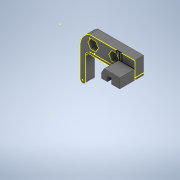
# Autodesk Inventor part: mount_battery
Saved by Autodesk Inventor 2022.2 (Build 262287000, 287)
## iProperties
Created: 2021-01-30
Part Number: mount_battery
Material: ABS Plastic
Document SubType Name: Modeling
Designer: User
Density: 1.06 g/cm^3
Appearance: Smooth - Black
Author: User
Autodesk Inventor part; units mm, degrees
ref_plane "YZ Plane" through (0, 0, 0) normal (1, 0, 0) x (0, 1, 0)
ref_plane "XZ Plane" through (0, 0, 0) normal (0, 1, 0) x (-1, 0, 0)
ref_plane "Work Plane1" through (0, 0, 0) normal (0, 0, 1) x (1, 0, 0)
sketch "mount_sketch" plane through (0, 0, 0) normal (0, 0, 1) x (1, 0, 0)
  circle A0 centre (42, 55.2584) radius 1.55 projected
  circle A1 centre (28, 55.2584) radius 1.55 projected
  line L0 (45, 60.2584) -> (25, 60.2584)
  line L1 (25, 60.2584) -> (15.4, 52.7584)
  line L2 (15.4, 52.7584) -> (15.4, 29.5584)
  line L3 (15.4, 29.5584) -> (19.4, 29.5584)
  line L4 (19.4, 29.5584) -> (19.4, 48.7584)
  line L5 (19.4, 48.7584) -> (23, 48.7584)
  circle A2 centre (42, -54.7416) radius 1.55 construction
  circle A3 centre (28, -54.7416) radius 1.55 construction
  line L6 (47, -54.627) -> (47, 66.2497) construction
  circle A4 centre (12, 51.2584) radius 1.55 construction
  circle A5 centre (12, -37.8416) radius 1.55 construction
  circle A6 centre (12, -54.7416) radius 1.55 construction
  circle A7 centre (29, -68.7416) radius 1.55 construction
  circle A8 centre (14, -68.7416) radius 1.55 construction
  line L7 (45, 50.2584) -> (25, 50.2584)
  line L8 (25, 50.2584) -> (23, 48.7584)
  line L9 (45, 60.2584) -> (46.5, 60.2584)
  line L10 (46.5, 60.2584) -> (46.5, 50.2584)
  line L11 (46.5, 50.2584) -> (45, 50.2584)
  line L12 (23, 48.7584) -> (23, 58.6959)
  line L13 (35, 55.2584) -> (35, 60.2584)
  line L14 (35, 55.2584) -> (35, 50.2584)
  line L15 (46.5, 60.2584) -> (50, 60.2584)
  line L16 (50, 60.2584) -> (50, 50.2584)
  line L17 (50, 50.2584) -> (46.5, 50.2584)
  line L18 (50, 60.2584) -> (56, 60.2584)
  line L19 (56, 60.2584) -> (56, 50.2584)
  line L20 (56, 50.2584) -> (50, 50.2584)
  line L21 (53, 50.2584) -> (56, 50.2584)
  line L22 (53, 50.2584) -> (53, 60.2584)
  point P0 (0, 0)
  dimension "d1" = 110
  dimension "d2" = 6.5
  dimension "d3" = 27.6
  dimension "d4" = 4
  dimension "d5" = 14
  dimension "d6" = 5
  dimension "d7" = 19.2
  dimension "d9" = 3.4
  dimension "d13" = 3
  dimension "d30" = 2
  dimension "d32" = 5
  dimension "d62" = 4.5
  dimension "d77" = 8
  dimension "d78" = 6
  constraints: 44 end point, 11 perpendicular, 4 horizontal, 4 midpoint, 2 vertical alignment, 1 collinear, 1 point on line, 1 vertical
  measures "d1" distance of A2.centre A0.centre
  measures "d2" distance from line of A0.centre L5
  measures "d3" distance between parallel lines of L6 L4
  measures "d4" distance between parallel lines of L4 L2
  measures "d5" vertical distance of A3.centre A7.centre
  measures "d6" distance from line of L0 A0.centre
  measures "d7" distance between parallel lines of L5 L3
  measures "d9" distance from line of L2 A4.centre
  measures "d13" horizontal distance of L0.end A1.centre
  measures "d30" horizontal distance of L0.end L5.end
  measures "d32" distance from line of L7 A0.centre
  measures "d62" distance from line of L10 A0.centre
  measures "d77" distance from line of L16 A0.centre
  measures "d78" distance of L19.end L16.end
extrude "mount" add sketch "mount_sketch" along normal blind 6 contours L9 L10 L11 L7 L14 L13 L0 | L13 L14 L7 L8 L12 L1 L0 | L12 L5 L4 L3 L2 L1
fillet "common" radius 2 2 edges at (25, 60.2584, 3) (25, 50.2584, 3)
sketch "nuts_sketch" plane through (0, 0, 6) normal (0, 0, 1) x (1, 0, 0)
  circle A0 centre (42, 55.2584) radius 1.55 projected
  circle A1 centre (28, 55.2584) radius 1.55 projected
  line L0 (38.4782, 55.2584) -> (40.2391, 58.3084)
  line L1 (40.2391, 58.3084) -> (43.7609, 58.3084)
  line L2 (43.7609, 58.3084) -> (45.5218, 55.2584)
  line L3 (45.5218, 55.2584) -> (43.7609, 52.2084)
  line L4 (43.7609, 52.2084) -> (40.2391, 52.2084)
  line L5 (40.2391, 52.2084) -> (38.4782, 55.2584)
  line L6 (31.5218, 55.2584) -> (29.7609, 52.2084)
  line L7 (29.7609, 52.2084) -> (26.2391, 52.2084)
  line L8 (26.2391, 52.2084) -> (24.4782, 55.2584)
  line L9 (24.4782, 55.2584) -> (26.2391, 58.3084)
  line L10 (26.2391, 58.3084) -> (29.7609, 58.3084)
  line L11 (29.7609, 58.3084) -> (31.5218, 55.2584)
  point P0 (0, 0)
  dimension "d26" = 6.1
  dimension "d27" = 6.1
  constraints: 24 end point, 2 coincident, 2 horizontal alignment, 26 other
  measures "d26" distance between parallel lines of L2 L5
  measures "d27" distance between parallel lines of L8 L11
extrude "nuts" cut sketch "nuts_sketch" against normal blind 3
sketch "Sketch11" plane through (25.6667, 50.2584, 0) normal (0, -1, 0) x (1, 0, 0)
  point P0 (-25.6667, 0)
  point P1 (12.8115, -12)
sketch "Sketch13" plane through (46.5, 50.2584, 0) normal (1, 0, 0) x (0, 0, -1)
  line L0 (0, 10) -> (-6, 10) projected
  line L1 (0, 0) -> (-6, 0) projected
  line L2 (-6, 10) -> (-6, 0)
  line L3 (0, 0) -> (0, 10) projected
  line L4 (-6, 0) -> (0, 0)
  line L5 (0, 0) -> (0, 10)
  line L6 (0, 10) -> (-6, 10)
  point P0 (0, -50.2584)
  constraints: 8 end point, 3 perpendicular, 1 vertical
extrude "Extrusion11" add sketch "Sketch13" along normal blind 9.5
sketch "Sketch20" plane through (19.4, 29.5584, 0) normal (1, 0, 0) x (0, 0, -1)
  line L0 (-6, 0) -> (-6, 19.2) projected
  line L1 (-6, 0) -> (-6, 19.2)
  line L2 (0, 19.2) -> (-6, 19.2) projected
  line L3 (-6, 19.2) -> (0, 19.2)
  line L4 (0, 0) -> (-6, 0) projected
  line L5 (0, 19.2) -> (0, 0)
  line L6 (0, 0) -> (-6, 0)
  point P0 (0, -29.5584)
  constraints: 8 end point, 2 collinear, 1 perpendicular, 1 vertical
extrude "Extrusion15" add sketch "Sketch20" along normal blind 3.6
sketch "Sketch21" plane through (0, 0, 6) normal (0, 0, 1) x (1, 0, 0)
  line L0 (15.4, 29.5584) -> (23, 29.5584) projected
  line L1 (19.2, 29.5584) -> (19.2, 55.7272)
  line L2 (24.4573, 59.8345) -> (15.4, 52.7584) projected
  line L3 (15.4, 52.7584) -> (15.4, 29.5584) projected
  line L4 (19.2, 29.5584) -> (15.4, 29.5584)
  line L5 (15.4, 29.5584) -> (15.4, 52.7584)
  line L6 (15.4, 52.7584) -> (19.2, 55.7272)
  line L7 (23, 48.7584) -> (24.4667, 49.8584) projected
  line L8 (23, 48.7584) -> (19.2, 48.7584)
  line L9 (23, 48.7584) -> (23, 29.5584) projected
  line L10 (23, 48.7584) -> (23, 58.6959)
  line L11 (19.2, 48.7584) -> (23, 58.6959)
  point P0 (0, 0)
  constraints: 14 end point, 3 point on line, 2 vertical, 1 collinear, 1 horizontal, 1 midpoint, 1 perpendicular
extrude "Extrusion16" cut sketch "Sketch21" against normal blind 6 contours L3 L2 L1 L0
sketch "Sketch22" plane through (0, 0, 6) normal (0, 0, 1) x (1, 0, 0)
  line L0 (23, 48.7584) -> (23, 29.5584) projected
  line L1 (23, 48.7584) -> (23, 58.6959)
  line L2 (24.4573, 59.8345) -> (19.2, 55.7272) projected
  line L3 (23, 48.7584) -> (19.2, 48.7584)
  line L4 (19.2, 29.5584) -> (19.2, 55.7272) projected
  point P0 (0, 0)
  constraints: 4 end point, 2 point on line, 1 perpendicular, 1 vertical
fillet "Fillet12" radius 10 1 edges at (19.2, 55.7272, 3)
fillet "Fillet13" radius 2 1 edges at (23, 48.7584, 3)
fillet "Fillet14" radius 2 2 edges at (23, 29.5584, 3) (19.2, 29.5584, 3)
sketch "Sketch27" plane through (25.6667, 50.2584, 0) normal (0, -1, 0) x (1, 0, 0)
  line L0 (0, 0) -> (0, 6) projected
  line L1 (0, 0) -> (30.3333, 0) projected
  line L2 (30.3333, 6) -> (30.3333, 0) projected
  line L3 (0, 6) -> (30.3333, 6) projected
  point P0 (-25.6667, 0)
extrude "Extrusion21" add sketch "Sketch27" along normal blind 1.5
sketch "Sketch28" plane through (25.6667, 48.7584, 0) normal (-1, 0, 0) x (0, 0, 1)
  line L0 (0, 1.5) -> (6, 1.5) projected
  line L1 (0, 1.5) -> (0, 0) projected
  line L2 (6, 0) -> (0, 0) projected
  line L3 (6, 1.5) -> (6, 0) projected
  point P0 (0, -48.7584)
extrude "Extrusion22" add sketch "Sketch28" along normal through all
fillet "Fillet19" radius 1 1 edges at (23.2679, 48.7584, 3)
sketch "Sketch29" plane through (0, 0, 6) normal (0, 0, 1) x (1, 0, 0)
  line L0 (24.4782, 55.2584) -> (26.2391, 58.3084) projected
  line L1 (26.2391, 58.3084) -> (29.7609, 58.3084) projected
  line L2 (29.7609, 58.3084) -> (31.5218, 55.2584) projected
  line L3 (31.5218, 55.2584) -> (29.7609, 52.2084) projected
  line L4 (29.7609, 52.2084) -> (26.2391, 52.2084) projected
  line L5 (26.2391, 52.2084) -> (24.4782, 55.2584) projected
  line L6 (45.5218, 55.2584) -> (43.7609, 52.2084) projected
  line L7 (43.7609, 52.2084) -> (40.2391, 52.2084) projected
  line L8 (40.2391, 52.2084) -> (38.4782, 55.2584) projected
  line L9 (38.4782, 55.2584) -> (40.2391, 58.3084) projected
  line L10 (40.2391, 58.3084) -> (43.7609, 58.3084) projected
  line L11 (43.7609, 58.3084) -> (45.5218, 55.2584) projected
  line L12 (19.2, 50.8497) -> (19.2, 31.5484) projected
  arc A0 (19.2, 31.5484) -> (21, 29.5584) centre (21.2, 31.5484) ccw projected
  arc A1 (21, 29.5584) -> (23, 31.5584) centre (21, 31.5584) ccw projected
  line L13 (23, 47.7584) -> (23, 31.5584) projected
  arc A2 (24, 48.7584) -> (23, 47.7584) centre (24, 47.7584) ccw projected
  line L14 (56, 48.7584) -> (24, 48.7584) projected
  line L15 (56, 60.2584) -> (56, 48.7584) projected
  line L16 (25.6886, 60.2584) -> (56, 60.2584) projected
  arc A3 (25.6886, 60.2584) -> (24.4573, 59.8345) centre (25.6886, 58.2584) ccw projected
  line L17 (24.4573, 59.8345) -> (23.0436, 58.73) projected
  arc A4 (23.0436, 58.73) -> (19.2, 50.8497) centre (29.2, 50.8497) ccw projected
  line L18 (45.5218, 55.2584) -> (56, 55.2584)
  line L19 (56, 60.2584) -> (56, 48.7584) projected
  line L20 (43.7609, 58.3084) -> (45.5218, 55.2584) projected
  line L21 (45.5218, 55.2584) -> (45.5218, 48.7584)
  line L22 (45.5218, 55.2584) -> (45.5218, 60.2584)
  line L23 (43.7609, 58.3084) -> (43.7609, 60.2584)
  line L24 (43.7609, 52.2084) -> (43.7609, 48.7584)
  line L25 (43.7609, 60.2584) -> (45.5218, 60.2584)
  line L26 (25.6886, 60.2584) -> (56, 60.2584) projected
  line L27 (45.5218, 60.2584) -> (47.2828, 60.2584)
  line L28 (47.2828, 60.2584) -> (47.2828, 48.7584)
  line L29 (45.5218, 55.2584) -> (43.7609, 52.2084) projected
  line L30 (43.7609, 52.2084) -> (56, 52.2084)
  line L31 (56, 60.2584) -> (56, 48.7584) projected
  point P0 (0, 0)
  constraints: 18 end point, 9 point on line, 5 perpendicular, 2 collinear, 1 horizontal
extrude "Extrusion24" add sketch "Sketch29" along normal blind 10 contours L21 L30 L6 | L18 L28 L30 L21 | L30 L21 L14 L24 | L18 L15 L30 L28 | L30 L28 L14 L21 | L30 L15 L14 L28
sketch "Sketch30" plane through (25.6667, 48.7584, 0) normal (0, -1, 0) x (1, 0, 0)
  line L0 (-1.6667, 0) -> (-1.6667, 6) projected
  line L1 (30.3333, 0) -> (-1.6667, 0) projected
  line L2 (30.3333, 0) -> (30.3333, 16) projected
  line L3 (18.0943, 6) -> (-1.6667, 6) projected
  line L4 (18.0943, 16) -> (30.3333, 16) projected
  line L5 (22, 16) -> (24.7, 16)
  line L6 (24.7, 16) -> (24.7, 3)
  line L7 (24.7, 3) -> (22, 3)
  line L8 (22, 3) -> (22, 16)
  line L9 (18.0943, 16) -> (30.3333, 16) projected
  line L10 (18.0943, 6) -> (18.0943, 16) projected
  point P0 (-25.6667, 0)
  dimension "d132" = 2.7
  constraints: 8 end point, 2 parallel, 1 horizontal, 1 perpendicular, 1 point on line
  measures "d132" distance of L6.end L7.end
extrude "Extrusion25" cut sketch "Sketch30" against normal blind 3.45 contours L6 L7 L8 L4
fillet "Fillet20" radius 1 1 edges at (49.0167, 52.2084, 3)
equation "\"d27\" = d26"
body "Solid1"
